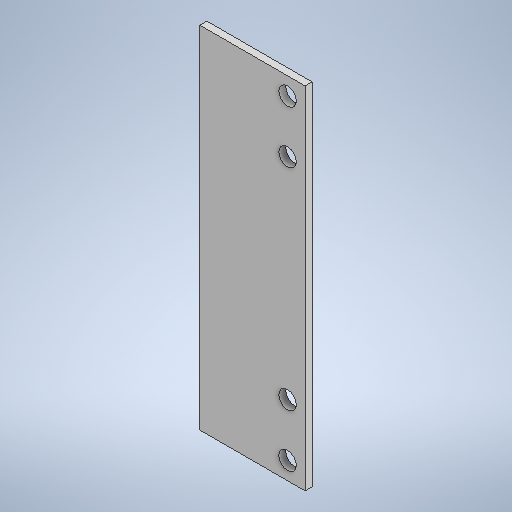
# Autodesk Inventor part: Ухо на швеллер пямое_CPY
Saved by Autodesk Inventor 2025 (Build 290162010, 162A)
## iProperties
Created: 2024-06-15
Part Number: Ухо на швеллер пямое_CPY
Material: Generic
Document SubType Name: Sheet Metal
Designer: admin
Density: 1 g/cm^3
Sheet Metal Rule: Default
Appearance: Default
Author: admin
Autodesk Inventor part; units mm, degrees
ref_plane "YZ Plane" through (0, 0, 0) normal (1, 0, 0) x (0, 1, 0)
ref_plane "XZ Plane" through (0, 0, 0) normal (0, 1, 0) x (-1, 0, 0)
ref_plane "XY Plane" through (0, 0, 0) normal (0, 0, 1) x (1, 0, 0)
sketch "Sketch1" plane through (0, 0, 0) normal (0, 1, 0) x (-1, 0, 0)
  line L0 (60, -200) -> (-60, -200)
  line L1 (-60, -200) -> (-60, 200)
  line L2 (-60, 200) -> (60, 200)
  line L3 (60, 200) -> (60, -200)
  line L4 (60, -200) -> (-60, 200) construction
  line L5 (-60, -200) -> (60, 200) construction
  point P0 (0, 0)
  point P1 (0, 0)
  dimension "d16" = 120
  dimension "d17" = 400
  measures "d16" distance of L1.end L2.end
  measures "d17" distance of L0.end L1.end
extrude "Plate1" add sketch "Sketch1" along normal blind 8
sketch "Sketch2" plane through (0, 0, 0) normal (0, -1, 0) x (1, 0, 0)
  line L0 (40, 180) -> (40, -180) construction
  line L1 (-60, -200) -> (60, -200) projected
  line L2 (60, -200) -> (60, 200) projected
  line L3 (60, 200) -> (-60, 200) projected
  line L4 (-60, 200) -> (-60, -200) projected
  point P0 (40, 0)
  point P1 (40, 0)
  point P2 (0, 0)
  point P3 (40, 120)
  point P4 (40, -120)
  dimension "d19" = 20
  dimension "d20" = 20
  dimension "d21" = 360
  dimension "d22" = 120
  dimension "d23" = 120
  constraints: 2 coincident, 2 end point, 2 point on line, 1 horizontal alignment, 1 midpoint, 1 vertical
  measures "d19" distance between parallel lines of L2 L0
  measures "d20" distance from line of L0.start L3
  measures "d21" distance of L0.start L0.end
  measures "d22" distance of point (40, 0) point (40, -120)
  measures "d23" distance of point (40, 0) point (40, 120)
hole "Hole1" at (40, 0, 180) at (40, 0, -180) at (40, 0, -120) at (40, 0, 120) direction (0, 1, 0) diameter 20 end through all
equation "\"d20\" = d19"
equation "\"d22\" = d23"
equation "\"d3\" = d19"
equation "\"d8\" = Thickness"
equation "\"d2\" = Thickness"
equation "\"BendRadius\" = Thickness"
equation "\"BendReliefWidth\" = Thickness"
equation "\"BendReliefDepth\" = 0.5 * Thickness"
equation "\"CornerReliefSize\" = 4 * Thickness"
equation "\"MinimumRemnant\" = 2 * Thickness"
equation "\"TransitionRadius\" = BendRadius"
equation "\"JacobiRadiusSize\" = BendRadius"
equation "\"GapSize\" = Thickness"
equation "\"Thickness\" = 8"
body "Solid1"
